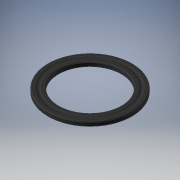
# Autodesk Inventor part: 51110 Housing washer
Saved by Autodesk Inventor 2019 (Build 230136000, 136)
## iProperties
Created: 2023-07-26
Part Number: 51110 Housing washer
Material: Generic
Catalog Web Link: www.cadenas.de
Description: With flat seet HW-
Vendor: NSK_RB
Document SubType Name: Modeling
Designer: psAdmin
Manufacturer: NSK_RB
Mass: 6.48689 g
Surface Area: 47.664 cm^2
Volume: 6.48689 cm^3
Density: 1 g/cm^3
Appearance: PSOLRGB-175-175-175
Category: PARTsolutions
Company: NSK_RB
Title: 51110 Housing washer
Author: Cadenas PARTsolutions
PSOL_IDENT_0: {$CADENAS_DATA/23d-libs/nsk_rb/roller_bearings/thrust_bearings/single_direction_tbb/with_flat_seet_h
PSOL_IDENT_1: w.prj},193 {VTYP=3D},{NB=51110 Housing washer},{LINA=51110 Housing washer},{NN=With flat seet HW},{D
PSOL_IDENT_2: ATE=27.09.2022 23:23:10},{GEOMDATE=23.08.2022 10:33:13},{VERSION=},{LINEID=6550},{WBVAR=},{WBNUMERIC=
PSOL_IDENT_3: }  {NB=51110 Housing washer},{LINA=51110 Housing washer},{KT=DUMMY},{N=18},{IDNR=},{STAN=},{NO=31},{
PSOL_IDENT_4: ORDER=51110},{SD=50},{D=70},{T=14},{T3=0.0},{T4=0},{SR=0.6},{CAN=29000},{COAN=75500},{CA=2960},{COA=
PSOL_IDENT_5: 7700},{GRE=3200},{OIL=4800},{SD1=70},{D1=52},{D2=0},{D3=0},{SB=0.0},{A=0.0},{R=0},{SDA=62},{DA=58},{
PSOL_IDENT_6: SRA=0.6},{MASS=0.153},{DIST=2.800}
NB: 51110 Housing washer
NN: With flat seet HW
NBSYN: $ORDER. Housing washer
LINA: 51110 Housing washer
CATALOG: NSK Rolling Bearing
N: 18
NO: 31
ORDER: 51110
SD: 50
D: 70
T: 14
T3: 0
T4: 0
SR: 0.6
CAN: 29000
COAN: 75500
CA: 2960
COA: 7700
GRE: 3200
OIL: 4800
SD1: 70
D1: 52
D2: 0
D3: 0
SB: 0
A: 0
R: 0
SDA: 62
DA: 58
SRA: 0.6
MASS: 0.153
SUPPLIER: NSK_RB
ARTICLENO: 51110 Housing washer
BOMINFO: 51110 Housing washer
CREATOR: CADENAS GmbH
Autodesk Inventor part; units mm, degrees
sketch "Sketch_1" plane through (0, 0, 0) normal (0, 0, 1) x (0, 1, 0)
  line L0 (3.8889, 0) -> (0, 0)
  arc A0 (0, 26.6) -> (0.6, 26) centre (0.6, 26.6) ccw
  line L1 (0.6, 26) -> (3.2889, 26)
  arc A1 (3.2889, 26) -> (3.8889, 26.6) centre (3.2889, 26.6) ccw
  line L2 (3.8889, 26.6) -> (3.8889, 28.8966)
  arc A2 (3.8889, 32.1034) -> (3.8889, 28.8966) centre (7, 30.5) ccw
  line L3 (3.8889, 32.1034) -> (3.8889, 34.4)
  arc A3 (3.8889, 34.4) -> (3.2889, 35) centre (3.2889, 34.4) ccw
  line L4 (3.2889, 35) -> (0.6, 35)
  arc A4 (0.6, 35) -> (0, 34.4) centre (0.6, 34.4) ccw
  line L5 (0, 34.4) -> (0, 26.6)
  constraints: 12 end point, 10 point on circle, 5 centre point
revolve "Revolution1" add sketch "Sketch_1" angle 360 about axis through (0, 3.8889, 0) along (0, 1, 0)
ref_plane "HW_B_1_XY" through (-30.5, 7, 0) normal (0, 1, 0) x (0, 0, -1)
ref_plane "HW_B_1_YZ" through (-30.5, 7, 0) normal (0, 0, -1) x (-1, 0, 0)
ref_plane "HW_B_1_ZX" through (-30.5, 7, 0) normal (-1, 0, 0) x (0, 1, 0)
ref_plane "HW_B_10_XY" through (30.5, 7, 0) normal (0, 1, 0) x (0, 0, -1)
ref_plane "HW_B_10_YZ" through (30.5, 7, 0) normal (0, 0, -1) x (-1, 0, 0)
ref_plane "HW_B_10_ZX" through (30.5, 7, 0) normal (-1, 0, 0) x (0, 1, 0)
ref_plane "HW_B_11_XY" through (28.6606, 7, -10.4316) normal (0, 1, 0) x (0, 0, -1)
ref_plane "HW_B_11_YZ" through (28.6606, 7, -10.4316) normal (0, 0, -1) x (-1, 0, 0)
ref_plane "HW_B_11_ZX" through (28.6606, 7, -10.4316) normal (-1, 0, 0) x (0, 1, 0)
ref_plane "HW_B_12_XY" through (23.3644, 7, -19.605) normal (0, 1, 0) x (0, 0, -1)
ref_plane "HW_B_12_YZ" through (23.3644, 7, -19.605) normal (0, 0, -1) x (-1, 0, 0)
ref_plane "HW_B_12_ZX" through (23.3644, 7, -19.605) normal (-1, 0, 0) x (0, 1, 0)
ref_plane "HW_B_13_XY" through (15.25, 7, -26.4138) normal (0, 1, 0) x (0, 0, -1)
ref_plane "HW_B_13_YZ" through (15.25, 7, -26.4138) normal (0, 0, -1) x (-1, 0, 0)
ref_plane "HW_B_13_ZX" through (15.25, 7, -26.4138) normal (-1, 0, 0) x (0, 1, 0)
ref_plane "HW_B_14_XY" through (5.2963, 7, -30.0366) normal (0, 1, 0) x (0, 0, -1)
ref_plane "HW_B_14_YZ" through (5.2963, 7, -30.0366) normal (0, 0, -1) x (-1, 0, 0)
ref_plane "HW_B_14_ZX" through (5.2963, 7, -30.0366) normal (-1, 0, 0) x (0, 1, 0)
ref_plane "HW_B_15_XY" through (-5.2963, 7, -30.0366) normal (0, 1, 0) x (0, 0, -1)
ref_plane "HW_B_15_YZ" through (-5.2963, 7, -30.0366) normal (0, 0, -1) x (-1, 0, 0)
ref_plane "HW_B_15_ZX" through (-5.2963, 7, -30.0366) normal (-1, 0, 0) x (0, 1, 0)
ref_plane "HW_B_16_XY" through (-15.25, 7, -26.4138) normal (0, 1, 0) x (0, 0, -1)
ref_plane "HW_B_16_YZ" through (-15.25, 7, -26.4138) normal (0, 0, -1) x (-1, 0, 0)
ref_plane "HW_B_16_ZX" through (-15.25, 7, -26.4138) normal (-1, 0, 0) x (0, 1, 0)
ref_plane "HW_B_17_XY" through (-23.3644, 7, -19.605) normal (0, 1, 0) x (0, 0, -1)
ref_plane "HW_B_17_YZ" through (-23.3644, 7, -19.605) normal (0, 0, -1) x (-1, 0, 0)
ref_plane "HW_B_17_ZX" through (-23.3644, 7, -19.605) normal (-1, 0, 0) x (0, 1, 0)
ref_plane "HW_B_18_XY" through (-28.6606, 7, -10.4316) normal (0, 1, 0) x (0, 0, -1)
ref_plane "HW_B_18_YZ" through (-28.6606, 7, -10.4316) normal (0, 0, -1) x (-1, 0, 0)
ref_plane "HW_B_18_ZX" through (-28.6606, 7, -10.4316) normal (-1, 0, 0) x (0, 1, 0)
ref_plane "HW_B_2_XY" through (-28.6606, 7, 10.4316) normal (0, 1, 0) x (0, 0, -1)
ref_plane "HW_B_2_YZ" through (-28.6606, 7, 10.4316) normal (0, 0, -1) x (-1, 0, 0)
ref_plane "HW_B_2_ZX" through (-28.6606, 7, 10.4316) normal (-1, 0, 0) x (0, 1, 0)
ref_plane "HW_B_3_XY" through (-23.3644, 7, 19.605) normal (0, 1, 0) x (0, 0, -1)
ref_plane "HW_B_3_YZ" through (-23.3644, 7, 19.605) normal (0, 0, -1) x (-1, 0, 0)
ref_plane "HW_B_3_ZX" through (-23.3644, 7, 19.605) normal (-1, 0, 0) x (0, 1, 0)
ref_plane "HW_B_4_XY" through (-15.25, 7, 26.4138) normal (0, 1, 0) x (0, 0, -1)
ref_plane "HW_B_4_YZ" through (-15.25, 7, 26.4138) normal (0, 0, -1) x (-1, 0, 0)
ref_plane "HW_B_4_ZX" through (-15.25, 7, 26.4138) normal (-1, 0, 0) x (0, 1, 0)
ref_plane "HW_B_5_XY" through (-5.2963, 7, 30.0366) normal (0, 1, 0) x (0, 0, -1)
ref_plane "HW_B_5_YZ" through (-5.2963, 7, 30.0366) normal (0, 0, -1) x (-1, 0, 0)
ref_plane "HW_B_5_ZX" through (-5.2963, 7, 30.0366) normal (-1, 0, 0) x (0, 1, 0)
ref_plane "HW_B_6_XY" through (5.2963, 7, 30.0366) normal (0, 1, 0) x (0, 0, -1)
ref_plane "HW_B_6_YZ" through (5.2963, 7, 30.0366) normal (0, 0, -1) x (-1, 0, 0)
ref_plane "HW_B_6_ZX" through (5.2963, 7, 30.0366) normal (-1, 0, 0) x (0, 1, 0)
ref_plane "HW_B_7_XY" through (15.25, 7, 26.4138) normal (0, 1, 0) x (0, 0, -1)
ref_plane "HW_B_7_YZ" through (15.25, 7, 26.4138) normal (0, 0, -1) x (-1, 0, 0)
ref_plane "HW_B_7_ZX" through (15.25, 7, 26.4138) normal (-1, 0, 0) x (0, 1, 0)
ref_plane "HW_B_8_XY" through (23.3644, 7, 19.605) normal (0, 1, 0) x (0, 0, -1)
ref_plane "HW_B_8_YZ" through (23.3644, 7, 19.605) normal (0, 0, -1) x (-1, 0, 0)
ref_plane "HW_B_8_ZX" through (23.3644, 7, 19.605) normal (-1, 0, 0) x (0, 1, 0)
ref_plane "HW_B_9_XY" through (28.6606, 7, 10.4316) normal (0, 1, 0) x (0, 0, -1)
ref_plane "HW_B_9_YZ" through (28.6606, 7, 10.4316) normal (0, 0, -1) x (-1, 0, 0)
ref_plane "HW_B_9_ZX" through (28.6606, 7, 10.4316) normal (-1, 0, 0) x (0, 1, 0)
ref_plane "HW_SW_XY" through (0, 0, 0) normal (0, 1, 0) x (0, 0, -1)
ref_plane "HW_SW_YZ" through (0, 0, 0) normal (0, 0, -1) x (-1, 0, 0)
ref_plane "HW_SW_ZX" through (0, 0, 0) normal (-1, 0, 0) x (0, 1, 0)
body "Solid1"
